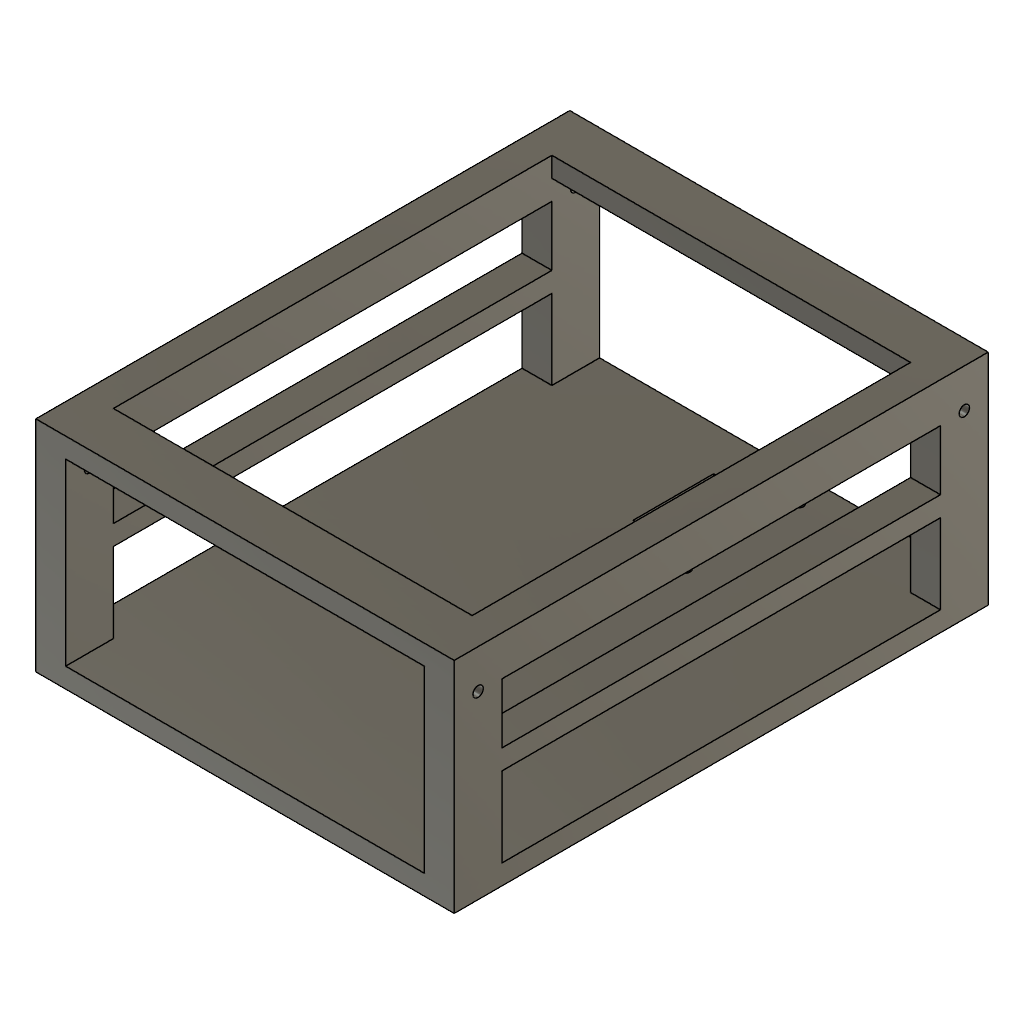
Upper_Card_Drop_Case (Autodesk Fusion 360 design; units mm, degrees)
Autodesk Fusion 360 part; units mm, degrees
sketch "Çizim1" plane through (0, 0, 0) normal (0, 0, 1) x (1, 0, 0)
  line L0 (52.5, 65) -> (-52.5, 65)
  line L1 (-52.5, 65) -> (-52.5, -65)
  line L2 (-52.5, -65) -> (52.5, -65)
  line L3 (52.5, -65) -> (52.5, 65)
  line L4 (52.5, 65) -> (-52.5, -65) construction
  line L5 (-52.5, 65) -> (52.5, -65) construction
  dimension "d1" = 105
  dimension "d2" = 130
  constraint horizontal L0
  constraint perpendicular L0 L1
  constraint parallel L0 L2
  constraint parallel L1 L3
  constraint coincident L4 origin
  constraint coincident L5 origin
  measures "d1" distance of L1.end L2.end
  measures "d2" distance of L0.end L1.end
extrude "Ekstrüzyon1" add sketch "Çizim1" against normal blind 5
sketch "Çizim2" plane through (0, 0, 0) normal (0, 0, 1) x (-1, 0, 0)
  line L0 (-52.5, 65) -> (-52.5, -65)
  line L1 (-52.5, -65) -> (52.5, -65)
  line L2 (52.5, -65) -> (52.5, 65)
  line L3 (52.5, 65) -> (-52.5, 65)
  line L4 (47.5, 60) -> (-47.5, 60)
  line L5 (-47.5, 60) -> (-47.5, -60)
  line L6 (-47.5, -60) -> (47.5, -60)
  line L7 (47.5, -60) -> (47.5, 60)
  dimension "d5" = -5
extrude "Ekstrüzyon2" add sketch "Çizim2" along normal blind 30
extrude "Ekstrüzyon3" add 1 faces at (-47.5, 20, 10) along direction (1, 0, 0) blind 2.5
extrude "Ekstrüzyon4" add 1 faces at (47.5, -20, 10) along direction (-1, 0, 0) blind 2.5
extrude "Ekstrüzyon5" add 1 faces at (-50, 20, 30) along direction (0, 0, 1) blind 20
extrude "Ekstrüzyon6" add 1 faces at (-17.5, -65, 13.3333) along direction (0, -1, 0) blind 2
extrude "Ekstrüzyon7" add 1 faces at (-17.5, 65, 31.6667) along direction (0, 1, 0) blind 2
sketch "Çizim4" plane through (52.5, 0, 0) normal (1, 0, 0) x (0, 1, 0)
  line L0 (-67, -5) -> (67, -5)
  line L1 (67, -5) -> (67, 50)
  line L2 (67, 50) -> (-67, 50)
  line L3 (-67, 50) -> (-67, -5)
  circle A0 centre (-61, 40.25) radius 1.3
  line L4 (0, 50) -> (0, -5)
  circle A1 centre (61, 40.25) radius 1.3
  dimension "d18" = 2.6
  dimension "d19" = 9.75
  dimension "d20" = 6
  constraint midpoint L2 L4.start
  constraint midpoint L0 L4.end
  constraint symmetric A0 L4 A1
  measures "d18" diameter of A0
  measures "d19" distance of L2 A0.centre
  measures "d20" distance of L3 A0.centre
extrude "Ekstrüzyon8" cut sketch "Çizim4" against normal blind 7.5 contours A0 | A1
extrude "Ekstrüzyon9" add 1 faces at (-15, 60, 29.8064) along direction (0, -1, 0) blind 5
extrude "Ekstrüzyon10" add 1 faces at (-15, -60, 29.8064) along direction (0, 1, 0) blind 5
mirror "Ayna1" about plane through (0, 0, 0) normal (1, 0, 0) of "Ekstrüzyon8"
sketch "Çizim5" plane through (-52.5, 0, 0) normal (-1, 0, 0) x (0, -1, 0)
  circle A0 centre (61, 40.25) radius 1.3
  circle A1 centre (-61, 40.25) radius 1.3
  line L0 (-67, -5) -> (67, -5)
  line L1 (67, -5) -> (67, 50)
  line L2 (67, 50) -> (-67, 50)
  line L3 (-67, 50) -> (-67, -5)
  line L4 (-55, 40) -> (-55, 25)
  line L5 (55, 40) -> (55, 25)
  line L6 (-55, 40) -> (55, 40)
  line L7 (55, 40) -> (55, 25)
  line L8 (55, 25) -> (-55, 25)
  line L9 (-55, 25) -> (-55, 40)
  dimension "d29" = 12
  dimension "d30" = 15
  dimension "d31" = 15
  dimension "d32" = 12
  dimension "d33" = 10
  constraint vertical L4
  constraint perpendicular L2 L5
  constraint horizontal L4.start L5.start
  constraint horizontal L6
  constraint vertical L7
  constraint horizontal L8
  constraint vertical L9
  measures "d29" distance of L3 L4
  measures "d30" distance of L4.start L4.end
  measures "d31" distance of L5.start L5.end
  measures "d32" distance of L1 L5
  measures "d33" distance of L2 L4.start
extrude "Ekstrüzyon11" cut sketch "Çizim5" against normal blind 105 contours L4 L5 L6 L7 L8 L9
sketch "Çizim6" plane through (-52.5, 0, 0) normal (-1, 0, 0) x (0, -1, 0)
  line L0 (55, 40) -> (55, 25)
  line L1 (55, 25) -> (-55, 25)
  line L2 (-55, 25) -> (-55, 40)
  line L3 (-55, 40) -> (55, 40)
  circle A0 centre (61, 40.25) radius 1.3
  circle A1 centre (-61, 40.25) radius 1.3
  line L4 (-67, -5) -> (67, -5)
  line L5 (67, -5) -> (67, 50)
  line L6 (67, 50) -> (-67, 50)
  line L7 (-67, 50) -> (-67, -5)
  line L8 (55, 25) -> (55, -5)
  line L9 (-55, 25) -> (-55, -5)
  line L10 (-55, 10) -> (55, 10)
  line L11 (-55, 20) -> (55, 20)
  line L12 (55, 20) -> (55, 0)
  line L13 (55, 0) -> (-55, 0)
  line L14 (-55, 0) -> (-55, 20)
  constraint coincident L0.end L1.start
  constraint perpendicular L1 L8
  constraint coincident L1.end L2.start
  constraint coincident L4 L9.end
  constraint perpendicular L4 L9
  constraint midpoint L9 L10.start
  constraint midpoint L8 L10.end
  constraint horizontal L11
  constraint vertical L12
  constraint horizontal L13
  constraint vertical L14
  constraint coincident L8 L12.end
  constraint coincident L9 L11.start
extrude "Ekstrüzyon12" cut sketch "Çizim6" against normal blind 105 contours L8 L9 L10 L11 L12 L14 | L8 L9 L10 L12 L13 L14
sketch "Çizim7" plane through (0, 67, 0) normal (0, 1, 0) x (-1, 0, 0)
  line L0 (-52.5, 50) -> (-52.5, -5)
  line L1 (-52.5, -5) -> (52.5, -5)
  line L2 (52.5, -5) -> (52.5, 50)
  line L3 (52.5, 50) -> (-52.5, 50)
  line L4 (-45, 50) -> (-45, -5)
  line L5 (45, 50) -> (45, -5)
  line L6 (-45, 45) -> (45, 45)
  line L7 (45, 45) -> (45, 0)
  line L8 (45, 0) -> (-45, 0)
  line L9 (-45, 0) -> (-45, 45)
  dimension "d38" = 7.5
  dimension "d39" = 7.5
  constraint coincident L3 L4.start
  constraint coincident L1 L4.end
  constraint perpendicular L1 L4
  constraint coincident L3 L5.start
  constraint coincident L1 L5.end
  constraint perpendicular L1 L5
  constraint horizontal L6
  constraint vertical L7
  constraint horizontal L8
  constraint vertical L9
  constraint coincident L5 L7.end
  constraint coincident L4 L6.start
  measures "d38" distance of L0 L4
  measures "d39" distance of L2 L5
extrude "Ekstrüzyon13" cut sketch "Çizim7" against normal blind 134 contours L4 L5 L6 L7 L8 L9
sketch "Çizim8" plane through (0, 0, -5) normal (0, 0, -1) x (1, 0, 0)
  line L0 (52.5, -67) -> (52.5, 67)
  line L1 (52.5, 67) -> (-52.5, 67)
  line L2 (-52.5, 67) -> (-52.5, -67)
  line L3 (-52.5, -67) -> (52.5, -67)
  line L4 (5.5, -35.9) -> (-5.5, -35.9)
  line L5 (-5.5, -35.9) -> (-5.5, -56.1)
  line L6 (-5.5, -56.1) -> (5.5, -56.1)
  line L7 (5.5, -56.1) -> (5.5, -35.9)
  line L8 (0, -35.9) -> (0, -56.1)
  circle A0 centre (11.6, -31.8) radius 1.3
  circle A1 centre (11.6, -60.2) radius 1.3
  line L9 (11.6, -31.8) -> (11.6, -33.1)
  line L10 (11.6, -31.8) -> (11.6, -33.1)
  line L11 (11.6, -58.9) -> (11.6, -60.2)
  line L12 (11.6, -31.8) -> (11.6, -60.2)
  line L13 (11.6, -46) -> (5.5, -46)
  point P0 (5.5, -46)
  dimension "d42" = 11
  dimension "d43" = 20.2
  dimension "d44" = 10.9
  dimension "d45" = 28.4
  dimension "d46" = 2.6
  dimension "d47" = 2.6
  dimension "d48" = 6.1
  constraint horizontal L4
  constraint vertical L5
  constraint horizontal L6
  constraint vertical L7
  constraint midpoint L4 L8.start
  constraint midpoint L6 L8.end
  constraint coincident origin L8
  constraint vertical L10
  constraint midpoint L7 P0
  constraint coincident A0.centre L9.start
  constraint coincident A1.centre L11.end
  constraint coincident A0 L9.end
  constraint coincident A1 L11.start
  constraint collinear L10 L11
  constraint midpoint L12 L13.start
  constraint coincident P0 L13.end
  constraint parallel L4 L13
  measures "d42" distance of L4.start L4.end
  measures "d43" distance of L4.start L6.end
  measures "d44" distance of L3 L6
  measures "d45" distance of A0.centre A1.centre
  measures "d46" diameter of A0
  measures "d47" diameter of A1
  measures "d48" distance of L7 L10
extrude "Ekstrüzyon14" cut sketch "Çizim8" against normal blind 5 contours L4 L6 L7 L8 | L4 L5 L6 L8 | A0 | A1
